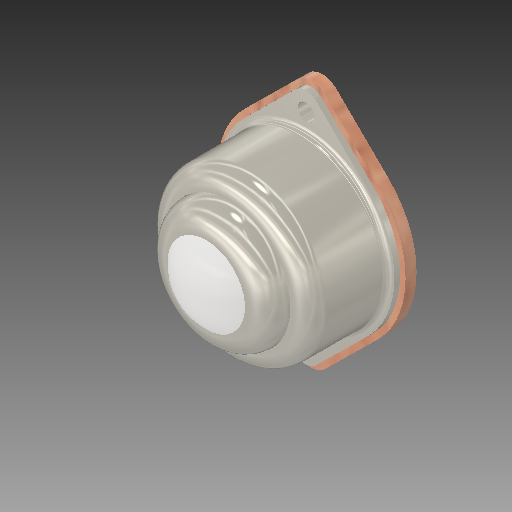
# Autodesk Inventor part: wheel2
Saved by Autodesk Inventor 2017 (Build 210142000, 142)
## iProperties
Created: 2019-10-24
Part Number: wheel2
Material: Generic
Document SubType Name: Modeling
Designer: User
Density: 1 g/cm^3
Appearance: Default
Mass: 13.8416 g
Surface Area: 37.2625 cm^2
Volume: 13.8416 cm^3
Author: User
Autodesk Inventor part; units mm, degrees
ref_plane "YZ Plane" through (0, 0, 0) normal (1, 0, 0) x (0, 1, 0)
ref_plane "XZ Plane" through (0, 0, 0) normal (0, 1, 0) x (-1, 0, 0)
ref_plane "XY Plane" through (0, 0, 0) normal (0, 0, 1) x (1, 0, 0)
sketch "Sketch1" plane through (0, 0, 0) normal (0, 0, 1) x (1, 0, 0)
  circle A0 centre (0, 0) radius 14.7
  dimension "d0" = 29.4
  constraints: 1 centre point, 1 coincident
  measures "d0" diameter of A0
extrude "Extrusion1" add sketch "Sketch1" along normal blind 14
sketch "Sketch2" plane through (0, 0, 14) normal (0, 0, 1) x (1, 0, 0)
  circle A0 centre (0, 0) radius 11.2
  dimension "d3" = 22.4
  constraints: 1 centre point, 1 coincident
  measures "d3" diameter of A0
extrude "Extrusion2" add sketch "Sketch2" along normal blind 4
fillet "Fillet1" radius 3.2 1 edges at (-14.7, 0, 14)
fillet "Fillet2" radius 4 1 edges at (-11.2, 0, 18)
sketch "Sketch3" plane through (0, 0, 0) normal (1, 0, 0) x (0, 1, 0)
  line L0 (-7.2, 18) -> (7.2, 18) projected
  line L1 (7.2, 18) -> (-7.2, 18)
  arc A0 (7, 18) -> (-7, 18) centre (0, 11.3333) ccw
  line L2 (0, 18) -> (0, 21)
  point P0 (0, 0)
  dimension "d9" = 14
  constraints: 4 end point, 3 point on circle, 2 point on line, 1 centre point, 1 horizontal, 1 midpoint
  measures "d9" distance of A0.start A0.end
revolve "Revolution1" add sketch "Sketch3" angle 360 about axis through (0, 0, 18) along (0, 0, 1) picked at (4.1722, 18.4238) contours L2 A0 L0
sketch "Sketch4" plane through (0, 0, 0) normal (0, 0, -1) x (-1, 0, 0)
  arc A0 (-1.7555, -20.7411) -> (1.7555, -20.7411) centre (0, -18.9612) ccw
  line L0 (1.7555, -20.7411) -> (11.2352, -11.3917)
  line L1 (-1.7555, -20.7411) -> (-11.2549, -11.3723)
  arc A1 (1.7361, 20.7603) -> (-1.7554, 20.7412) centre (0.0001, 18.9613) ccw
  line L2 (1.7361, 20.7603) -> (11.2352, 11.3917)
  line L3 (-1.7554, 20.7412) -> (-11.2549, 11.3723)
  arc A2 (-11.2352, 11.3917) -> (-11.2352, -11.3917) centre (0, 0) ccw
  arc A3 (11.2352, -11.3917) -> (11.2352, 11.3917) centre (0, 0) ccw
  circle A4 centre (0, 18) radius 1.5
  circle A5 centre (0, -18) radius 1.5
  dimension "d13" = 5
  dimension "d19" = 32
  dimension "d22" = 3
  dimension "d23" = 3
  constraints: 8 end point, 8 point on circle, 6 centre point, 5 tangent, 2 point on line, 1 coincident
  measures "d13" diameter of A0
  measures "d19" distance between parallel lines of L0 L3
  measures "d22" diameter of A4
  measures "d23" diameter of A5
sketch "Sketch5" plane through (0, 0, 0) normal (0, 1, 0) x (-1, 0, 0)
  point P0 (0, 0)
extrude "Extrusion4" add sketch "Sketch4" along normal blind 1
fillet "Fillet5" radius 1 1 edges at (-14.7, 0, 0)
sketch "Sketch7" plane through (0, 0, -1) normal (0, 0, -1) x (-1, 0, 0)
  line L0 (-11.2352, -11.3917) -> (-1.7555, -20.7411) projected
  line L1 (1.7555, -20.7411) -> (11.2352, -11.3917) projected
  arc A0 (-1.7555, -20.7411) -> (1.7555, -20.7411) centre (0, -18.9612) ccw projected
  arc A1 (-11.2352, 11.3917) -> (-11.2352, -11.3917) centre (0, 0) ccw projected
  line L2 (-1.7554, 20.7412) -> (-11.2352, 11.3917) projected
  line L3 (11.2352, 11.3917) -> (1.7361, 20.7603) projected
  circle A2 centre (0, -18) radius 1.5 projected
  circle A3 centre (0, 18) radius 1.5 projected
  arc A4 (-1.7555, -20.7411) -> (1.7555, -20.7411) centre (0, -18.9612) ccw projected
  line L4 (1.7555, -20.7411) -> (11.2352, -11.3917) projected
  arc A5 (11.2352, -11.3917) -> (11.2352, 11.3917) centre (0, 0) ccw projected
  line L5 (11.2352, 11.3917) -> (1.7361, 20.7603) projected
  arc A6 (1.7361, 20.7603) -> (-1.7554, 20.7412) centre (0.0001, 18.9613) ccw projected
  line L6 (-1.7554, 20.7412) -> (-11.2352, 11.3917) projected
  arc A7 (-11.2352, 11.3917) -> (-11.2352, -11.3917) centre (0, 0) ccw projected
  line L7 (-11.2352, -11.3917) -> (-1.7555, -20.7411) projected
  arc A8 (1.7361, 20.7603) -> (-1.7554, 20.7412) centre (0.0001, 18.9613) ccw projected
  arc A9 (11.9374, -12.1037) -> (11.9374, 12.1037) centre (0, 0) ccw
  line L8 (11.9374, -12.1037) -> (2.4577, -21.4531)
  arc A10 (-2.4577, -21.4531) -> (2.4577, -21.4531) centre (0, -18.9612) ccw
  line L9 (-2.4577, -21.4531) -> (-11.9374, -12.1037)
  arc A11 (-11.9374, 12.1037) -> (-11.9374, -12.1037) centre (0, 0) ccw
  line L10 (-11.9374, 12.1037) -> (-2.4576, 21.4532)
  arc A12 (2.4347, 21.4758) -> (-2.4576, 21.4532) centre (0.0001, 18.9613) ccw
  line L11 (2.4347, 21.4758) -> (11.9374, 12.1037)
  dimension "d27" = 1
  constraints: 8 end point, 8 point on circle, 4 centre point, 7 other
  measures "d27" radial gap between concentric circles of A5 A9
extrude "Extrusion5" add sketch "Sketch7" along normal blind 2 contours A1 L2 A6 L3 A5 L1 A0 L0 | L8 A10 L9 A11 L10 A12 L11 A9
body "Solid1"
